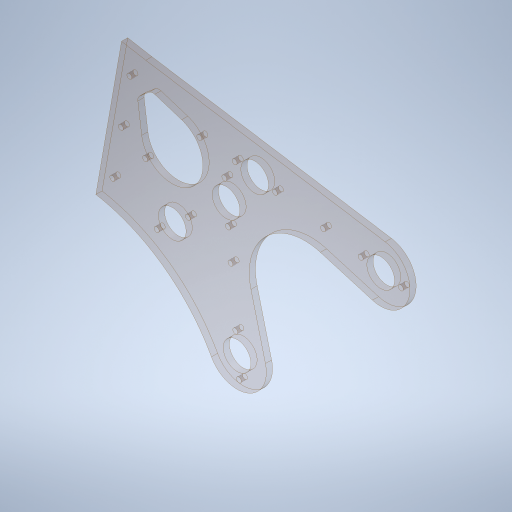
# Autodesk Inventor part: GP9-002
Saved by Autodesk Inventor 2023.4 (Build 274418000, 418)
## iProperties
Created: 2025-02-24
Part Number: GP9-002
Material: Polycarbonate, Smoke
Document SubType Name: Modeling
Designer: dlangdon
Density: 1.2 g/cm^3
Appearance: Polycarbonate - Smoked
Author: dlangdon
Autodesk Inventor part; units mm, degrees
ref_plane "YZ Plane" through (0, 0, 0) normal (1, 0, 0) x (0, 1, 0)
ref_plane "XZ Plane" through (0, 0, 0) normal (0, 1, 0) x (-1, 0, 0)
ref_plane "XY Plane" through (0, 0, 0) normal (0, 0, 1) x (1, 0, 0)
sketch "Sketch1" plane through (0, 0, 0) normal (0, 0, 1) x (1, 0, 0)
  circle A0 centre (74.0871, 74.0871) radius 50.8 construction
  circle A1 centre (-74.0871, -74.0871) radius 50.8 construction
  circle A2 centre (0, 0) radius 53.975 construction
  line L0 (-38.1661, -38.1661) -> (38.1661, 38.1661) construction
  line L1 (74.0871, 74.0871) -> (-74.0871, -74.0871) construction
  line L2 (-4.3707, 6.2419) -> (-4.3707, 53.7978) construction
  line L3 (-229.1249, -124.8871) -> (636.2672, -124.8871) construction
  circle A3 centre (145.5955, -67.7371) radius 57.15 construction
  circle A4 centre (74.0871, 74.0871) radius 14.2875
  circle A5 centre (-74.0871, -74.0871) radius 14.2875
  circle A6 centre (-4.3707, 6.2419) radius 57.15 construction
  circle A7 centre (-74.0871, -74.0871) radius 30.1625 construction
  circle A8 centre (74.0871, 74.0871) radius 30.1625 construction
  circle A9 centre (-55.9252, 94.4505) radius 14.2875
  line L4 (-55.9252, 94.4505) -> (74.0871, 74.0871) construction
  circle A10 centre (74.0871, 74.0871) radius 14.3256 construction
  circle A11 centre (-74.0871, -74.0871) radius 14.3256 construction
  circle A12 centre (-85.4337, 57.0202) radius 14.2875
  line L5 (-74.0871, -74.0871) -> (-85.4337, 57.0202) construction
  circle A13 centre (-85.4337, 57.0202) radius 23.8316 construction
  circle A14 centre (-55.9252, 94.4505) radius 23.8316 construction
  line L6 (11.8393, 61.0449) -> (65.5319, 45.1633)
  line L7 (-44.8488, -66.678) -> (-59.7696, -7.7964)
  arc A15 (11.8393, 61.0449) -> (-59.7696, -7.7964) centre (-4.3707, 6.2419) ccw
  line L8 (-193.3057, 147.0275) -> (-168.2916, 142.6169)
  line L9 (-168.2916, 142.6169) -> (-194.7556, -7.4679) construction
  line L10 (-194.7556, -7.4679) -> (-219.7697, -3.0572) construction
  line L11 (-219.7697, -3.0572) -> (-193.3057, 147.0275) construction
  line L12 (-236.345, -97.0603) -> (32.8251, -144.5223) construction
  line L13 (-188.895, 172.0416) -> (169.2102, 108.898) construction
  line L14 (-188.895, 172.0416) -> (-236.345, -97.0603) construction
  circle A16 centre (-141.0504, 77.7003) radius 31.75
  line L15 (-83.3789, 33.2774) -> (-78.4672, -23.4763) construction
  circle A17 centre (14.4887, 83.4218) radius 9.525 construction
  line L16 (-180.7986, 144.8222) -> (-207.2626, -5.2625) construction
  line L17 (-185.2093, 119.8081) -> (-202.8519, 19.7516) construction
  circle A18 centre (-141.0504, 77.7003) radius 17.4625 construction
  circle A19 centre (-141.0504, 77.7003) radius 9.525
  circle A20 centre (-55.9252, 94.4505) radius 30.1816 construction
  line L18 (-193.3057, 147.0275) -> (-219.7697, -3.0572)
  arc A21 (65.5319, 45.1633) -> (78.7588, 103.8856) centre (74.0871, 74.0871) ccw
  arc A22 (-100.544, -88.5718) -> (-44.8488, -66.678) centre (-74.0871, -74.0871) ccw
  line L19 (-141.0504, 77.7003) -> (-127.6733, 88.925) construction
  line L20 (-113.0802, 101.1701) -> (-169.0206, 54.2305) construction
  circle A23 centre (-169.0206, 54.2305) radius 4.7625 construction
  line L21 (0, 0) -> (-4.3707, 6.2419) construction
  circle A24 centre (74.0871, 74.0871) radius 28.6512 construction
  line L22 (66.5905, 46.434) -> (-59.6635, 80.6607) construction
  line L23 (75.4045, 102.708) -> (-55.2683, 108.7228) construction
  line L24 (-168.2916, 142.6169) -> (78.7588, 103.8856)
  line L25 (-141.0504, 77.7003) -> (-140.9896, 10.4919) construction
  circle A25 centre (-140.9896, 10.4919) radius 31.75 construction
  circle A26 centre (-140.9896, 10.4919) radius 14.2875
  line L26 (-85.4337, 57.0202) -> (-140.9896, 10.4919) construction
  circle A27 centre (-141.0504, 77.7003) radius 25.4 construction
  arc A28 (-100.544, -88.5718) -> (-219.7697, -3.0572) centre (-249.1988, -169.9579) ccw
  point P0 (-80.923, 4.9006)
  point P1 (-194.0306, 69.7798)
  point P2 (-194.0306, 69.7798)
  point P3 (-144.0827, 94.8975)
  point P4 (-157.4597, 83.6728)
  point P5 (-154.4274, 66.4756)
  point P6 (-138.018, 60.5031)
  point P7 (-124.641, 71.7278)
  point P8 (-121.5928, 94.0271)
  point P9 (-145.461, 102.7144)
  point P10 (-164.9186, 86.3876)
  point P11 (-160.5079, 61.3735)
  point P12 (-136.6397, 52.6862)
  point P13 (-117.1822, 69.013)
  dimension "d7" = 101.6
  dimension "d18" = 47.6631
  dimension "d34" = 34.925
  dimension "d65" = 50.8
  dimension "d3" = 45
  dimension "d4" = 0
  dimension "d8" = 107.95
  dimension "d9" = 28.575
  dimension "d10" = 101.6
  dimension "d11" = 114.3
  dimension "d12" = 114.3
  dimension "d13" = 15.875
  dimension "d14" = 15.875
  dimension "d15" = 131.5974
  dimension "d16" = 28.6512
  dimension "d17" = 131.5974
  dimension "d19" = 47.6631
  dimension "d22" = 25.4
  dimension "d23" = 152.4
  dimension "d26" = 273.2533
  dimension "d27" = 63.5
  dimension "d30" = 190.5
  dimension "d31" = 10
  dimension "d32" = 19.05
  dimension "d33" = 101.6
  dimension "d35" = 19.05
  dimension "d36" = 6.35
  dimension "d40" = 360
  dimension "d44" = 9.525
  dimension "d55" = 80
  dimension "d56" = 7.62
  dimension "d57" = 25.4
  dimension "d58" = 57.3024
  dimension "d59" = 63.5
  dimension "d60" = 67.2084
  dimension "d61" = 72.4662
  dimension "d62" = 55
  dimension "d68" = 360
  dimension "d70" = 38.1
  dimension "d71" = 40
  constraints: 54 end point, 25 centre point, 23 coincident, 21 point on circle, 17 tangent, 7 midpoint, 5 equal radius, 5 point on line, 4 collinear, 4 parallel, 2 horizontal, 1 concentric, 1 perpendicular, 1 vertical, 29 other
  measures "d3" angle of L2 L0
  measures "d4" distance between parallel lines of L0 L1
  measures "d8" diameter of A2
  measures "d9" diameter of A4
  measures "d10" diameter of A0
  measures "d11" diameter of A3
  measures "d12" diameter of A6
  measures "d13" radial gap between concentric circles of A5 A7
  measures "d14" radial gap between concentric circles of A4 A8
  measures "d15" distance of L4.start L4.end
  measures "d16" diameter of A10
  measures "d17" distance of L5.start L5.end
  measures "d19" diameter of A14
  measures "d22" distance of L9.end L10.end
  measures "d23" distance of L10.end L8.start
  measures "d26" distance of L13.start L12.start
  measures "d27" diameter of A16
  measures "d30" distance from line of point (0, 0) L9
  measures "d31" angle of L3 L12
  measures "d32" diameter of A17
  measures "d33" distance of L17.start L17.end
  measures "d35" diameter of A19
  measures "d36" radial gap between concentric circles of A14 A20
  measures "d44" diameter of A23
  measures "d55" angle of L1 L21
  measures "d56" distance of L21.start L21.end
  measures "d57" distance between parallel lines of L13 L8
  measures "d58" diameter of A24
  measures "d59" diameter of A25
  measures "d60" distance of L19.start L25.end
  measures "d61" distance of L26.start L26.end
  measures "d62" angle of L15 L26
  measures "d70" distance from line of L9 L19.start
  measures "d71" angle of L9 L20
extrude "Extrusion1" add sketch "Sketch1" along normal blind 6.35 contours A15 L7 A22 A28 L18 L8 L24 A21 L6
hole "Hole1" at (14.4887, 83.4218, 0) at (-185.2093, 119.8081, 0) at (-194.0306, 69.7798, 0) at (-202.8519, 19.7516, 0) at (-127.6733, 88.925, 0) at (-144.0827, 94.8975, 0) at (-157.4597, 83.6728, 0) at (-154.4274, 66.4756, 0) at (-138.018, 60.5031, 0) at (-124.641, 71.7278, 0) at (-113.0802, 101.1701, 0) at (-169.0206, 54.2305, 0) at (-136.6397, 52.6862, 0) at (-160.5079, 61.3735, 0) at (-164.9186, 86.3876, 0) at (-145.461, 102.7144, 0) at (-121.5928, 94.0271, 0) at (-117.1822, 69.013, 0) at (-80.923, 4.9006, 0) direction (0, 0, 1) diameter 5.1054 end through all clearance for "Flat Head Machine Screw (82)" size "#10" standard "Ansi Unified Screw Threads"
sketch "Sketch2" plane through (0, 0, 6.35) normal (0, 0, 1) x (1, 0, 0)
  circle A0 centre (-169.0206, 54.2305) radius 2.5527 construction
  circle A1 centre (-202.8519, 19.7516) radius 2.5527 construction
  circle A2 centre (-185.2093, 119.8081) radius 2.5527 construction
  circle A3 centre (14.4887, 83.4218) radius 2.5527 construction
  circle A4 centre (-194.0306, 69.7798) radius 2.5527 construction
  circle A5 centre (-113.0802, 101.1701) radius 2.5527 construction
  circle A6 centre (-80.923, 4.9006) radius 2.5527 construction
  line L0 (-44.8488, -66.678) -> (-59.7696, -7.7964) construction
  arc A7 (11.8393, 61.0449) -> (-59.7696, -7.7964) centre (-4.3707, 6.2419) ccw construction
  line L1 (11.8393, 61.0449) -> (65.5319, 45.1633) construction
  arc A8 (65.5319, 45.1633) -> (78.7588, 103.8856) centre (74.0871, 74.0871) ccw construction
  line L2 (78.7588, 103.8856) -> (-168.2916, 142.6169) construction
  line L3 (-168.2916, 142.6169) -> (-193.3057, 147.0275) construction
  line L4 (-193.3057, 147.0275) -> (-219.7697, -3.0572) construction
  arc A9 (-100.544, -88.5718) -> (-219.7697, -3.0572) centre (-249.1988, -169.9579) ccw construction
  arc A10 (-100.544, -88.5718) -> (-44.8488, -66.678) centre (-74.0871, -74.0871) ccw construction
  circle A11 centre (-85.4337, 57.0202) radius 14.2875 construction
  circle A12 centre (-140.9896, 10.4919) radius 14.2875 construction
  circle A13 centre (-55.9252, 94.4505) radius 14.2875 construction
  circle A14 centre (-74.0871, -74.0871) radius 14.2875 construction
  circle A15 centre (74.0871, 74.0871) radius 14.2875 construction
  line L5 (-75.8994, -53.1469) -> (-72.2749, -95.0273) construction
  line L6 (-157.1034, -3.0034) -> (-124.8759, 23.9872) construction
  line L7 (-87.2459, 77.9604) -> (-83.6214, 36.08) construction
  line L8 (-76.6906, 97.7029) -> (-35.1599, 91.1981) construction
  line L9 (53.3218, 77.3395) -> (94.8525, 70.8347) construction
  circle A16 centre (-85.4337, 57.0202) radius 14.2875 construction
  line L10 (-55.9252, 94.4505) -> (-85.4337, 57.0202) construction
  line L11 (-55.9252, 94.4505) -> (74.0871, 74.0871) construction
  line L12 (-85.4337, 57.0202) -> (-140.9896, 10.4919) construction
  line L13 (-85.4337, 57.0202) -> (-74.0871, -74.0871) construction
  point P0 (0, 0)
  point P1 (-85.4337, 57.0202)
  dimension "d72" = 42.037
  constraints: 19 end point, 14 coincident, 5 collinear, 5 midpoint, 4 equal length
  measures "d72" distance of L5.start L5.end
hole "Hole2" at (-75.8994, -53.1469, 6.35) at (-124.8759, 23.9872, 6.35) at (-72.2749, -95.0273, 6.35) at (-157.1034, -3.0034, 6.35) at (-83.6214, 36.08, 6.35) at (-87.2459, 77.9604, 6.35) at (-35.1599, 91.1981, 6.35) at (-76.6906, 97.7029, 6.35) at (94.8525, 70.8347, 6.35) at (53.3218, 77.3395, 6.35) direction (0, 0, -1) diameter 5.1054 end through all clearance for "Flat Head Machine Screw (82)" size "#10" standard "Ansi Unified Screw Threads"
sketch "Sketch3" plane through (0, 0, 6.35) normal (0, 0, 1) x (1, 0, 0)
  circle A0 centre (-141.0504, 77.7003) radius 31.75 projected
  line L0 (-172.5071, 73.3948) -> (-176.9188, 105.6284)
  line L1 (-176.9188, 105.6284) -> (-162.3257, 117.8735)
  line L2 (-162.3257, 117.8735) -> (-131.3479, 107.9315)
  circle A1 centre (-113.0802, 101.1701) radius 2.5527 projected
  circle A2 centre (-169.0206, 54.2305) radius 2.5527 projected
  line L3 (-113.0802, 101.1701) -> (-169.0206, 54.2305) construction
  line L4 (-169.0206, 54.2305) -> (-141.0504, 77.7003)
  line L5 (-141.0504, 77.7003) -> (-169.6223, 111.751) construction
  point P0 (0, 0)
  dimension "d80" = 44.45
  dimension "d82" = 19.05
  constraints: 12 end point, 2 point on circle, 2 tangent, 1 collinear, 1 equal length, 1 midpoint, 1 perpendicular
  measures "d80" distance from line of L4.end L1
  measures "d82" distance of L0.end L1.end
extrude "Extrusion2" cut sketch "Sketch3" against normal through all contours A0 L0 L1 L2
fillet "Fillet1" radius 6.35 2 edges at (-176.9188, 105.6284, 3.175) (-162.3257, 117.8735, 3.175)
body "Solid1"
